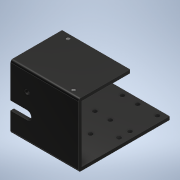
# Autodesk Inventor part: gantry
Saved by Autodesk Inventor 2020.2 (Build 242310000, 310)
## iProperties
Created: 2017-10-28
Part Number: gantry
Material: Ogólny
Document SubType Name: Modeling
Designer: wojte
Density: 1 g/cm^3
Appearance: Domyślna
Author: wojte
Autodesk Inventor part; units mm, degrees
note: some values were not read from the file. Chosen so that the rebuilt part matches the saved one: direction of "Otwór2".
ref_plane "YZ Plane" through (0, 0, 0) normal (1, 0, 0) x (0, 1, 0)
ref_plane "XZ Plane" through (0, 0, 0) normal (0, 1, 0) x (-1, 0, 0)
ref_plane "XY Plane" through (0, 0, 0) normal (0, 0, 1) x (1, 0, 0)
sketch "Szkic1" plane through (0, 0, 0) normal (0, 0, 1) x (1, 0, 0)
  line L0 (0, 80) -> (62, 80)
  line L1 (62, 80) -> (62, 0)
  line L2 (62, 0) -> (0, 0)
  line L3 (0, 0) -> (0, 80)
  point P0 (0, 0)
  dimension "d0" = 80
  dimension "d1" = 62
  constraints: 8 end point, 2 parallel, 1 coincident, 1 horizontal, 1 perpendicular
  measures "d0" distance of L0.end L1.end
  measures "d1" distance of L1.end L2.end
extrude "Wyciągnięcie proste1" add sketch "Szkic1" along normal blind 3
sketch "Szkic2" plane through (0, 0, 3) normal (0, 0, 1) x (1, 0, 0)
  line L0 (0, 80) -> (0, 0) projected
  line L1 (62, 80) -> (0, 80) projected
  line L2 (31, 80) -> (31, 0) construction
  line L3 (0, 0) -> (62, 0) projected
  line L4 (56, 75) -> (56, 50) construction
  line L5 (56, 62.5) -> (62, 62.5) construction
  line L6 (40, 30) -> (40, 5) construction
  line L7 (40, 17.5) -> (62.4441, 17.5) construction
  point P0 (6, 75)
  point P1 (24, 75)
  point P2 (24, 50)
  point P3 (6, 50)
  point P4 (38, 50)
  point P5 (38, 75)
  point P6 (22, 30)
  point P7 (22, 5)
  dimension "d4" = 18
  dimension "d5" = 25
  dimension "d6" = 6
  dimension "d7" = 5
  dimension "d10" = 32
  dimension "d15" = 18
  dimension "d16" = 25
  dimension "d17" = 45
  constraints: 10 end point, 4 horizontal alignment, 4 midpoint, 4 vertical alignment, 3 horizontal, 2 vertical, 1 symmetric about line, 4 other
  measures "d4" distance of point (24, 75) point (6, 75)
  measures "d5" distance of point (6, 50) point (6, 75)
  measures "d6" distance from line of L0 point (6, 75)
  measures "d7" distance from line of point (6, 75) L1
  measures "d10" distance of point (6, 50) point (38, 50)
  measures "d15" distance of L6.start point (22, 30)
  measures "d16" distance of L6.end L6.start
  measures "d17" distance between parallel lines of L7 L5
hole "Otwór1" at (6, 75, 3) at (24, 75, 3) at (24, 50, 3) at (6, 50, 3) at (38, 50, 3) at (56, 50, 3) at (56, 75, 3) at (38, 75, 3) at (22, 30, 3) at (40, 30, 3) at (40, 5, 3) at (22, 5, 3) direction (0, 0, -1) diameter 4 end through all
sketch "Szkic3" plane through (0, 0, 0) normal (0, -1, 0) x (1, 0, 0)
  line L0 (0, 0) -> (62, 0)
  line L1 (62, 0) -> (62, 55)
  line L2 (62, 55) -> (0, 55)
  line L3 (0, 55) -> (0, 0)
  line L4 (62, 0) -> (62, 3) projected
  point P0 (62, 1.5)
  dimension "d25" = 55
  constraints: 8 end point, 2 parallel, 1 horizontal, 1 midpoint, 1 perpendicular, 1 point on line
  measures "d25" distance of L2.end L0.start
extrude "Wyciągnięcie proste2" add sketch "Szkic3" along normal blind 3
sketch "Szkic4" plane through (0, 0, 55) normal (0, 0, 1) x (1, 0, 0)
  line L0 (62, 80) -> (62, -3) projected
  line L1 (62, -3) -> (0, -3)
  line L2 (0, -3) -> (0, 44)
  line L3 (0, 44) -> (62, 44)
  line L4 (62, 44) -> (62, -3)
  line L5 (0, 0) -> (0, -3) projected
  point P0 (0, -1.5)
  dimension "d28" = 47
  constraints: 8 end point, 2 parallel, 1 horizontal, 1 midpoint, 1 perpendicular, 1 point on line
  measures "d28" distance of L1.end L2.end
extrude "Wyciągnięcie proste3" add sketch "Szkic4" along normal blind 3
sketch "Szkic5" plane through (0, 0, 0) normal (0, 0, -1) x (-1, 0, 0)
  line L0 (0, -3) -> (-62, -3) projected
  line L1 (0, -3) -> (0, 80) projected
  line L2 (-31, -3) -> (-31, 80) construction
  line L3 (-62, 80) -> (0, 80) projected
  point P0 (0, 0)
  point P1 (-6, 40)
  point P2 (-56, 40)
  dimension "d31" = 43
  dimension "d32" = 6
  constraints: 2 end point, 2 midpoint, 1 horizontal alignment, 1 symmetric about line
  measures "d31" distance from line of L0 point (-6, 40)
  measures "d32" distance from line of L1 point (-6, 40)
hole "Otwór2" at (6, 40, 0) at (56, 40, 0) direction (0, 0, 1) diameter 4 end up to surface
thread "Gwint1" size "M4x0.7" class "6H" standard "ANSI Metric M Profile" full length
thread "Gwint2" size "M4x0.7" class "6H" standard "ANSI Metric M Profile" full length
thread "Gwint3" size "M4x0.7" class "6H" standard "ANSI Metric M Profile" full length
thread "Gwint4" size "M4x0.7" class "6H" standard "ANSI Metric M Profile" full length
thread "Gwint5" size "M4x0.7" class "6H" standard "ANSI Metric M Profile" full length
thread "Gwint6" size "M4x0.7" class "6H" standard "ANSI Metric M Profile" full length
thread "Gwint7" size "M4x0.7" class "6H" standard "ANSI Metric M Profile" full length
thread "Gwint8" size "M4x0.7" class "6H" standard "ANSI Metric M Profile" full length
thread "Gwint9" size "M4x0.7" class "6H" standard "ANSI Metric M Profile" full length
thread "Gwint10" size "M4x0.7" class "6H" standard "ANSI Metric M Profile" full length
thread "Gwint11" size "M4x0.7" class "6H" standard "ANSI Metric M Profile" full length
thread "Gwint12" size "M4x0.7" class "6H" standard "ANSI Metric M Profile" full length
thread "Gwint13" size "M4x0.7" class "6H" standard "ANSI Metric M Profile" full length
thread "Gwint14" size "M4x0.7" class "6H" standard "ANSI Metric M Profile" full length
sketch "Szkic6" plane through (0, 0, 0) normal (0, 1, 0) x (1, 0, 0)
  line L0 (0, -18) -> (19, -18)
  line L1 (19, -18) -> (19, -26)
  line L2 (19, -26) -> (0, -26)
  line L3 (0, -26) -> (0, -18)
  line L4 (62, -3) -> (0, -3) projected
  point P0 (0, 0)
  dimension "d68" = 15
  dimension "d69" = 8
  dimension "d70" = 19
  constraints: 8 end point, 2 parallel, 1 horizontal, 1 perpendicular, 1 vertical alignment
  measures "d68" distance between parallel lines of L0 L4
  measures "d69" distance of L0.end L1.end
  measures "d70" distance of L1.end L2.end
extrude "Wyciągnięcie proste4" cut sketch "Szkic6" against normal through all
full round fillet "Zaokrąglenie1" first side at (6.3333, -1, 18) centre faces at (19, -1, 20.6667) second side at (6.3333, -2, 26)
sketch "Szkic7" plane through (0, -3, 0) normal (0, -1, 0) x (1, 0, 0)
  line L0 (0, 58) -> (62, 58) projected
  line L1 (0, 26) -> (0, 58) projected
  point P0 (0, 0)
  point P1 (15, 40)
  dimension "d73" = 18
  dimension "d74" = 15
  measures "d73" distance from line of point (15, 40) L0
  measures "d74" distance from line of L1 point (15, 40)
hole "Otwór3" at (15, -3, 40) direction (0, 1, 0) diameter 4 end through all
fillet "Zaokrąglenie2" radius 2 2 edges at (31, -3, 58) (31, -3, 0)
sketch "Szkic8" plane through (0, 0, 58) normal (0, 0, 1) x (1, 0, 0)
  line L0 (62, 44) -> (0, 44) projected
  line L1 (31, 44) -> (31, 0) construction
  line L2 (62, 0) -> (0, 0) projected
  line L3 (0, 80) -> (0, 0) projected
  point P0 (9.5, 40)
  point P1 (52.5, 2)
  dimension "d83" = 43
  dimension "d84" = 38
  dimension "d85" = 21.5
  dimension "d86" = 4
  constraints: 2 end point, 2 midpoint
  measures "d83" horizontal distance of point (52.5, 2) point (9.5, 40)
  measures "d84" vertical distance of point (52.5, 2) point (9.5, 40)
  measures "d85" distance from line of L1 point (9.5, 40)
  measures "d86" distance from line of L0 point (9.5, 40)
hole "Otwór4" at (9.5, 40, 58) at (52.5, 2, 58) direction (0, 0, -1) diameter 3 depth 8 tip angle 118
